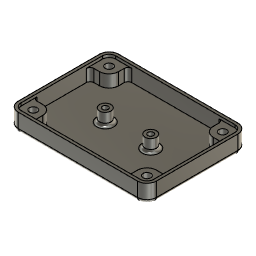
ATMega328P-AU Bootloader Burn Base (Autodesk Fusion 360 design; units mm, degrees)
Autodesk Fusion 360 part; units mm, degrees
sketch "Base Sketch" plane through (0, 0, 0) normal (0, 0, 1) x (1, 0, 0) in component "ATMega328P-AU Bootloader Burn Base"
  line L0 (0, 0) -> (73, 0)
  line L1 (73, 0) -> (73, 53)
  line L2 (73, 53) -> (0, 53)
  line L3 (0, 53) -> (0, 0)
  dimension "d1" = 73
  dimension "d2" = 53
  constraint horizontal L0
  constraint vertical L1
  constraint horizontal L2
  constraint vertical L3
  constraint coincident L0.start L3.end
  measures "d1" distance of L0.start L0.end
  measures "d2" distance of L0.start L2.end
extrude "Extrude1" add sketch "Base Sketch" along normal blind 9.5 in component "ATMega328P-AU Bootloader Burn Base"
fillet "Fillet1" radius 5 4 edges at (0, 0, 4.75) (73, 0, 4.75) (73, 53, 4.75) (0, 53, 4.75) in component "ATMega328P-AU Bootloader Burn Base"
shell "Shell1" thickness 1.5 removed faces 1 at (47, 17.6667, 9.5) in component "ATMega328P-AU Bootloader Burn Base"
fillet "Fillet6" radius 2 8 edges at (73, 26.5, 0) (71.5355, 51.5355, 0) (36.5, 53, 0) (1.4645, 51.5355, 0) (0, 26.5, 0) (1.4645, 1.4645, 0) (36.5, 0, 0) (71.5355, 1.4645, 0) in component "ATMega328P-AU Bootloader Burn Base"
sketch "Mounting Holes" plane through (0, 0, 1.5) normal (0, 0, 1) x (-1, 0, 0) in component "ATMega328P-AU Bootloader Burn Base"
  arc A0 (-5, -51.5) -> (-1.5, -48) centre (-5, -48) ccw
  line L0 (-1.5, -48) -> (-1.5, -5)
  arc A1 (-1.5, -5) -> (-5, -1.5) centre (-5, -5) ccw
  line L1 (-5, -1.5) -> (-68, -1.5)
  arc A2 (-68, -1.5) -> (-71.5, -5) centre (-68, -5) ccw
  line L2 (-71.5, -5) -> (-71.5, -48)
  arc A3 (-71.5, -48) -> (-68, -51.5) centre (-68, -48) ccw
  line L3 (-68, -51.5) -> (-5, -51.5)
  line L4 (-5, -1.5) -> (-68, -1.5)
  line L5 (-71.5, -5) -> (-71.5, -48)
  arc A4 (-68, -1.5) -> (-71.5, -5) centre (-68, -5) ccw
  line L6 (-1.5, -48) -> (-1.5, -5)
  arc A5 (-5, -51.5) -> (-1.5, -48) centre (-5, -48) ccw
  line L7 (-68, -51.5) -> (-5, -51.5)
  arc A6 (-71.5, -48) -> (-68, -51.5) centre (-68, -48) ccw
  line L8 (-1.5, -26.5) -> (-71.5, -26.5) construction
  line L9 (-36.5, -1.5) -> (-36.5, -51.5) construction
  line L10 (-48.5, -1.5) -> (-48.5, -51.5) construction
  line L11 (-24.5, -1.5) -> (-24.5, -51.5) construction
  circle A7 centre (-24.5, -26.5) radius 3
  circle A8 centre (-24.5, -26.5) radius 1.5
  circle A9 centre (-48.5, -26.5) radius 3
  circle A10 centre (-48.5, -26.5) radius 1.5
  line L12 (-1.5, -6.5) -> (-71.5, -6.5) construction
  line L13 (-6.5, -1.5) -> (-6.5, -51.5) construction
  circle A11 centre (-6.5, -6.5) radius 2.05
  line L14 (-11.5, -6.5) -> (-11.5, -1.5)
  line L15 (-6.5, -11.5) -> (-1.5, -11.5)
  arc A12 (-11.5, -6.5) -> (-6.5, -11.5) centre (-6.5, -6.5) ccw
  line L16 (-5, -1.5) -> (-11.5, -1.5)
  line L17 (-1.5, -5) -> (-1.5, -11.5)
  line L18 (-11.5, -46.5) -> (-11.5, -51.5)
  arc A13 (-6.5, -41.5) -> (-11.5, -46.5) centre (-6.5, -46.5) ccw
  line L19 (-6.5, -41.5) -> (-1.5, -41.5)
  circle A14 centre (-6.5, -46.5) radius 2.05
  line L20 (-1.5, -48) -> (-1.5, -41.5)
  line L21 (-5, -51.5) -> (-11.5, -51.5)
  circle A15 centre (-66.5, -6.5) radius 2.05
  circle A16 centre (-66.5, -46.5) radius 2.05
  line L22 (-5, -1.5) -> (-5, -51.5) construction
  line L23 (-1.5, -5) -> (-71.5, -5) construction
  arc A17 (-1.5, -5) -> (-5, -1.5) centre (-5, -5) ccw
  arc A18 (-5, -51.5) -> (-1.5, -48) centre (-5, -48) ccw
  line L24 (-71.5, -48) -> (-71.5, -41.5)
  line L25 (-66.5, -41.5) -> (-71.5, -41.5)
  arc A19 (-61.5, -46.5) -> (-66.5, -41.5) centre (-66.5, -46.5) ccw
  line L26 (-61.5, -46.5) -> (-61.5, -51.5)
  line L27 (-68, -51.5) -> (-61.5, -51.5)
  arc A20 (-71.5, -48) -> (-68, -51.5) centre (-68, -48) ccw
  line L28 (-71.5, -5) -> (-71.5, -11.5)
  arc A21 (-68, -1.5) -> (-71.5, -5) centre (-68, -5) ccw
  line L29 (-68, -1.5) -> (-61.5, -1.5)
  line L30 (-61.5, -6.5) -> (-61.5, -1.5)
  arc A22 (-66.5, -11.5) -> (-61.5, -6.5) centre (-66.5, -6.5) ccw
  line L31 (-66.5, -11.5) -> (-71.5, -11.5)
  dimension "d41" = 23
  dimension "d42" = 23
  dimension "d43" = 6
  dimension "d44" = 3
  dimension "d60" = 5
  dimension "d61" = 5
  dimension "d62" = 4.1
  constraint midpoint L6 L8.start
  constraint midpoint L5 L8.end
  constraint midpoint L4 L9.start
  constraint midpoint L7 L9.end
  constraint coincident L4 L10.start
  constraint coincident L7 L10.end
  constraint perpendicular L7 L10
  constraint coincident L4 L11.start
  constraint coincident L7 L11.end
  constraint perpendicular L7 L11
  constraint midpoint L11 A7.centre
  constraint concentric A7 A8
  constraint symmetric L9 A7 A9
  constraint symmetric L9 A8 A10
  constraint coincident L6 L12.start
  constraint coincident L5 L12.end
  constraint perpendicular L5 L12
  constraint coincident L4 L13.start
  constraint coincident L3 L13.end
  constraint perpendicular L3 L13
  constraint coincident L13 A11.centre
  constraint coincident L12 A11.centre
  constraint concentric A11 A12
  constraint coincident L12.start A12
  constraint coincident L12 L14.start
  constraint coincident L1 L14.end
  constraint tangent L14 A12
  constraint coincident L13 L15.start
  constraint coincident L6 L15.end
  constraint tangent L15 A12
  constraint coincident A1.end L1.start
  constraint coincident L0.end A1.start
  constraint symmetric L8 A11 A14
  constraint symmetric L8 L14.start L18.start
  constraint symmetric L8 L14.end L18.end
  constraint symmetric L8 L15.start A13.start
  constraint symmetric L8 L15.end L19.end
  constraint symmetric L8 A12 A13
  constraint symmetric L8 A1.end A0.start
  constraint symmetric L8 L0.end A0.end
  constraint symmetric L9 A11 A15
  constraint symmetric L9 A14 A16
  constraint coincident A2.end L2.start
  constraint symmetric L0.end L8 A0.end
  constraint symmetric A1.end L8 A0.start
  constraint symmetric L8 A17 A18
  constraint symmetric L0.end L9 A2.end
  constraint symmetric A1.end L9 L1.end
  constraint symmetric L9 L14.start L30.start
  constraint symmetric L9 L14.end L29.end
  constraint symmetric L9 L15.start A22.start
  constraint symmetric L9 L15.end L28.end
  constraint symmetric L9 A12 A22
  constraint symmetric L9 A1.end L1.end
  constraint symmetric L9 L0.end A2.end
  constraint symmetric L9 L18.start A19.start
  constraint symmetric L9 L18.end L26.end
  constraint symmetric L9 A13.start L25.start
  constraint symmetric L9 A13 A19
  constraint symmetric L9 L19.end L24.end
  constraint symmetric L9 A0.end L2.end
  constraint symmetric L9 A0.start A3.end
  constraint symmetric L9 A17 A21
  constraint symmetric L9 A18 A20
  measures "d41" distance of L2 L10
  measures "d42" distance of L6 L11
  measures "d43" diameter of A7
  measures "d44" diameter of A8
  measures "d60" distance of L0 L13
  measures "d61" distance of L4 L12
  measures "d62" diameter of A11
extrude "Extrude5" add sketch "Mounting Holes" along normal blind 6.5 contours A0 L0 L3 L6 A5 L7 L18 A13 L19 L20 L21 A18 | L2 A3 L3 L5 L7 A6 L24 L25 A19 L26 L27 A20 | L0 A1 L1 L4 L6 L14 L15 A12 L16 L17 A17 | L1 A2 L2 L4 L5 A4 L28 A21 L29 L30 A22 L31 | A7 | A9 in component "ATMega328P-AU Bootloader Burn Base"
fillet "Fillet11" radius 1.5 2 edges at (51.297, 25.4152, 1.5) (27.297, 25.4152, 1.5) in component "ATMega328P-AU Bootloader Burn Base"
fillet "Fillet12" radius 2 8 edges at (11.5, 1.5, 4.75) (1.5, 11.5, 4.75) (1.5, 41.5, 4.75) (11.5, 51.5, 4.75) (61.5, 51.5, 4.75) (71.5, 41.5, 4.75) (71.5, 11.5, 4.75) (61.5, 1.5, 4.75) in component "ATMega328P-AU Bootloader Burn Base"
component "ATMega328P-AU Bootloader Burn Base" placed x (1, 0, 0) y (0, 1, 0) z (0, 0, 1) at (0, 0, 0)
named bodies: "ESP32 Breakout Base"
